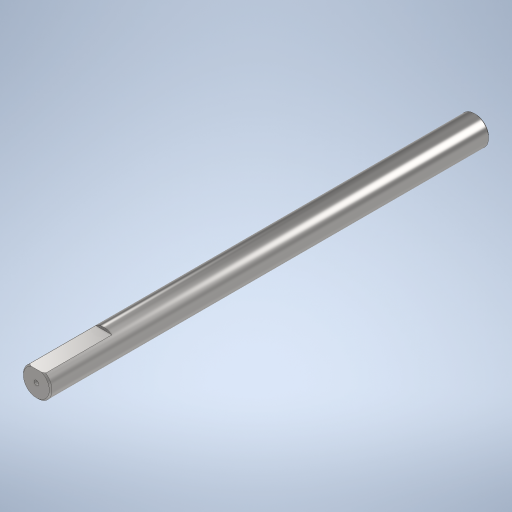
# Autodesk Inventor part: motorAxis
Saved by Autodesk Inventor 2023 (Build 270158000, 158)
## iProperties
Created: 2024-02-07
Part Number: motorAxis
Material: Stainless Steel
Document SubType Name: Modeling
Designer: victo
Density: 8 g/cm^3
Appearance: Semi-Polished
Author: victo
Autodesk Inventor part; units mm, degrees
ref_plane "YZ Plane" through (0, 0, 0) normal (1, 0, 0) x (0, 1, 0)
ref_plane "XZ Plane" through (0, 0, 0) normal (0, 1, 0) x (-1, 0, 0)
ref_plane "XY Plane" through (0, 0, 0) normal (0, 0, 1) x (1, 0, 0)
sketch "Sketch1" plane through (0, 0, 0) normal (0, 0, 1) x (1, 0, 0)
  circle A0 centre (0, 0) radius 3.175
  dimension "d0" = 6.35
  constraints: 1 centre point, 1 coincident
  measures "d0" diameter of A0
extrude "Extrusion1" add sketch "Sketch1" along normal blind 97.6
chamfer "Chamfer1" distance 0.3 angle 45 2 edges at (-3.175, 0, 97.6) (-3.175, 0, 0)
sketch "Sketch2" plane through (0, 0, 97.6) normal (0, 0, 1) x (1, 0, 0)
  circle A0 centre (0, 0) radius 0.5
  dimension "d6" = 1
  constraints: 1 centre point, 1 coincident
  measures "d6" diameter of A0
extrude "Extrusion2" cut sketch "Sketch2" against normal blind 2
sketch "Sketch3" plane through (0, 0, 0) normal (0, 0, -1) x (-1, 0, 0)
  circle A0 centre (0, 0) radius 0.5 projected
extrude "Extrusion3" cut sketch "Sketch3" against normal blind 2
sketch "Sketch4" plane through (0, 0, 97.6) normal (0, 0, 1) x (1, 0, 0)
  circle A0 centre (0, 0) radius 3.175 projected
  line L0 (-1.7861, 2.625) -> (-1.675, 2.625)
  line L1 (-1.675, 2.625) -> (1.7861, 2.625)
  dimension "d11" = 2.625
  constraints: 4 end point, 2 point on circle, 1 horizontal, 1 point on line
  measures "d11" distance from line of point (0, 0) L1
extrude "Extrusion4" cut sketch "Sketch4" against normal blind 15 contours L1 L0 A0 picked at (0.4083, 2.7411)
body "Solid1"
